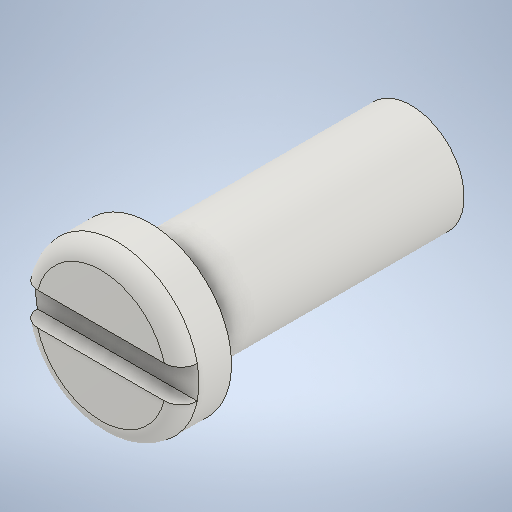
# Autodesk Inventor part: 17B - Crosshead Pin2
Saved by Autodesk Inventor 2025.2 (Build 292293000, 293)
## iProperties
Created: 2025-06-19
Part Number: 17B - Crosshead Pin2
Material: Steel AISI 1020 107 HR
Document SubType Name: Modeling
Designer: bless
Density: 7.87 g/cm^3
Appearance: Steel
Author: bless
Autodesk Inventor part; units mm, degrees
ref_plane "YZ Plane" through (0, 0, 0) normal (1, 0, 0) x (0, 1, 0)
ref_plane "XZ Plane" through (0, 0, 0) normal (0, 1, 0) x (-1, 0, 0)
ref_plane "XY Plane" through (0, 0, 0) normal (0, 0, 1) x (1, 0, 0)
sketch "Sketch1" plane through (0, 0, 0) normal (0, 0, 1) x (1, 0, 0)
  circle A0 centre (0, 0) radius 5
  dimension "d0" = 10
  constraints: 1 centre point, 1 coincident
  measures "d0" diameter of A0
extrude "Extrusion1" add sketch "Sketch1" along normal blind 3
sketch "Sketch2" plane through (0, 0, 3) normal (0, 0, 1) x (1, 0, 0)
  circle A0 centre (0, 0) radius 5 projected
  line L0 (-5.1933, 1) -> (5.1933, 1)
  line L1 (5.1933, 1) -> (5.1933, -1)
  line L2 (5.1933, -1) -> (-5.1933, -1)
  line L3 (-5.1933, -1) -> (-5.1933, 1)
  line L4 (-5.1933, 1) -> (5.1933, -1) construction
  line L5 (5.1933, 1) -> (-5.1933, -1) construction
  point P0 (-4.899, -1)
  point P1 (4.899, -1)
  point P2 (4.899, 1)
  point P3 (-4.899, 1)
  dimension "d3" = 2
  dimension "d4" = 79.101
  constraints: 12 end point, 2 midpoint, 2 parallel, 1 horizontal, 1 perpendicular
  measures "d3" distance of L0.end L1.end
  measures "d4" angle of L4 L1
extrude "Extrusion2" cut sketch "Sketch2" against normal blind 1 contours A0 L2 L0
fillet "Fillet1" radius 1 2 edges at (0, 5, 3) (0, -5, 3)
sketch "Sketch3" plane through (0, 0, 0) normal (0, 0, -1) x (-1, 0, 0)
  circle A0 centre (0, 0) radius 5 projected
  circle A1 centre (0, 0) radius 3.25
  dimension "d8" = 6.5
  constraints: 1 centre point, 1 coincident
  measures "d8" diameter of A1
extrude "Extrusion3" add sketch "Sketch3" along normal blind 16 contours A1
sketch "Sketch4" plane through (0, 0, -16) normal (0, 0, -1) x (-1, 0, 0)
  circle A0 centre (0, 0) radius 3.25 projected
  constraints: 1 coincident
hole "Hole1" at (0, 0, -16) direction (0, 0, 1) diameter 3.242 depth 8 tip angle 118 thread size "M4x0.7" class "6H" standard "ANSI Metric M Profile"
body "Solid1"
